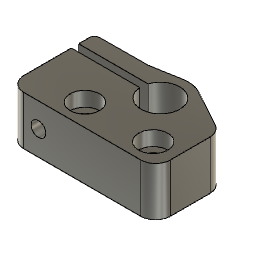
Y Axis Guide Rail Clamps (Autodesk Fusion 360 design; units mm, degrees)
Autodesk Fusion 360 part; units mm, degrees
sketch "Sketch4" plane through (0, 0, 0) normal (0, 0, 1) x (1, 0, 0)
  line L0 (-17.0224, 4.5069) -> (-7.2135, 4.5755)
  line L1 (-6.882, 4.6055) -> (-0.9889, 5.6389)
  line L2 (-18, 0) -> (-17.9997, 1.25) construction
  line L3 (-17.9997, 1.25) -> (-18.0154, 3.5)
  line L4 (-18, 0) -> (-18, -0.25) construction
  line L5 (-18, -0.25) -> (-3.9671, -0.25)
  line L6 (-17.9997, 1.25) -> (-3.7746, 1.2463)
  arc A0 (2.7555, 5.0182) -> (-0.9889, 5.6389) centre (0, 0) ccw
  arc A1 (-3.9671, -0.25) -> (-3.7746, 1.2463) centre (0, 0) ccw
  line L7 (-18, -0.25) -> (-18, -10)
  line L8 (-15, -13) -> (9, -13)
  line L9 (12, -10) -> (12, -1.8332)
  line L10 (10.444, 0.7965) -> (2.7555, 5.0182)
  arc A2 (-7.2135, 4.5755) -> (-6.882, 4.6055) centre (-7.2274, 6.5754) ccw
  arc A3 (-7.2135, 4.5755) -> (-6.882, 4.6055) centre (-7.2274, 6.5754) ccw
  arc A4 (12, -1.8332) -> (10.444, 0.7965) centre (9, -1.8332) ccw
  arc A5 (9, -13) -> (12, -10) centre (9, -10) ccw
  arc A6 (-18, -10) -> (-15, -13) centre (-15, -10) ccw
  arc A7 (-17.0224, 4.5069) -> (-18.0154, 3.5) centre (-17.0154, 3.507) ccw
  point P0 (-18.0224, 4.4999)
  dimension "d18" = 7.95
  dimension "d22" = 18
  dimension "d24" = 4.5
  dimension "d26" = 1.25
  dimension "d27" = 0.25
  dimension "d28" = 2
  dimension "d29" = 3
  dimension "d30" = 3
  dimension "d31" = 1
  dimension "d56" = 1.75
  constraint coincident A0.centre A1.centre
  constraint tangent L1 A0
  constraint perpendicular L0 L3
  constraint vertical L4
  constraint perpendicular L4 L5
  constraint perpendicular L2 L6
  constraint concentric A0 A1
  constraint tangent A0 L10
  constraint tangent L0 A2
  constraint tangent L1 A2
  constraint coincident L0 A2.start
  constraint coincident L1 A2.end
  constraint tangent L0 A3
  constraint tangent L1 A3
  constraint equal A2 A3
  constraint tangent L10 A4
  constraint tangent L9 A4
  constraint tangent L9 A5
  constraint tangent L8 A5
  constraint tangent L7 A6
  constraint tangent L8 A6
  constraint equal A5 A6
  constraint coincident P0 L3
  constraint coincident P0 L0
  constraint tangent L3 A7
  constraint tangent L0 A7
  measures "d18" diameter of A1
  measures "d22" distance of A0.centre L2.start
  measures "d24" distance of L2.start P0
  measures "d26" distance of L2.start L2.end
  measures "d27" distance of L2.start L4.end
  measures "d28" radius of A2
  measures "d29" radius of A4
  measures "d30" radius of A5
  measures "d31" radius of A7
  measures "d56" distance of A0 A1
extrude "Extrude2" add sketch "Sketch4" along normal blind 10 makes body 1
sketch "Sketch5" plane through (-0.0323, 4.6256, 0) normal (-0.006986, 0.999976, 0) x (-0.999976, -0.006986, 0)
  line L0 (7.1813, 0) -> (16.9905, 0)
  line L1 (16.9905, 0) -> (16.9905, 10)
  line L2 (16.9905, 10) -> (7.1813, 10)
  line L3 (7.1813, 10) -> (7.1813, 0)
  line L4 (12.0859, 10) -> (12.0859, 0) construction
  line L5 (16.9905, 5) -> (7.1813, 5) construction
  constraint midpoint L2 L4.start
  constraint midpoint L0 L4.end
  constraint midpoint L1 L5.start
  constraint midpoint L3 L5.end
hole "Hole2" at (-12.1179, 4.5412, 5) direction (0.006986, -0.999976, 0) diameter 3 end through all counterbore diameter 6 counterbore depth 2 bodies 1
sketch "Sketch6" plane through (0, 0, 10) normal (0, 0, 1) x (-1, 0, 0)
  line L0 (7.2135, -4.5755) -> (17.0224, -4.5069)
  arc A0 (17.0224, -4.5069) -> (18.0154, -3.5) centre (17.0154, -3.507) ccw
  line L1 (18.0154, -3.5) -> (17.9997, -1.25)
  line L2 (17.9997, -1.25) -> (3.7746, -1.2463)
  arc A1 (3.9671, 0.25) -> (3.7746, -1.2463) centre (0, 0) ccw
  line L3 (3.9671, 0.25) -> (18, 0.25)
  line L4 (18, 0.25) -> (18, 10)
  arc A2 (18, 10) -> (15, 13) centre (15, 10) ccw
  line L5 (15, 13) -> (-9, 13)
  arc A3 (-9, 13) -> (-12, 10) centre (-9, 10) ccw
  line L6 (-12, 10) -> (-12, 1.8332)
  arc A4 (-12, 1.8332) -> (-10.444, -0.7965) centre (-9, 1.8332) ccw
  line L7 (-10.444, -0.7965) -> (-2.7555, -5.0182)
  arc A5 (-2.7555, -5.0182) -> (0.9889, -5.6389) centre (0, 0) ccw
  line L8 (0.9889, -5.6389) -> (6.882, -4.6055)
  arc A6 (7.2135, -4.5755) -> (6.882, -4.6055) centre (7.2274, -6.5754) ccw
  line L9 (0, 0) -> (0, 3.975) construction
  line L10 (0, 3.975) -> (-12, 3.975) construction
  line L11 (-12, 3.975) -> (-12, 12.975) construction
  line L12 (-12, 8.475) -> (18, 8.475) construction
  line L13 (0, 3.975) -> (0, 13) construction
  line L14 (7, 8.475) -> (7, 6.4233) construction
  point P0 (-7, 8.475)
  point P1 (7, 8.475)
  dimension "d39" = 9
  dimension "d54" = 14
  dimension "d55" = 7
  constraint vertical L9
  constraint coincident A1.centre A5.centre
  constraint coincident L6 L10.end
  constraint tangent A1 L10
  constraint perpendicular L6 L10
  constraint perpendicular L10 L11
  constraint midpoint L11 L12.start
  constraint coincident L4 L12.end
  constraint perpendicular L4 L12
  constraint coincident L12 P0
  constraint coincident L12 P1
  constraint coincident L5 L13.end
  constraint perpendicular L5 L13
  constraint coincident P1 L14.start
  constraint perpendicular L12 L14
  measures "d39" distance of L10.end L11.end
  measures "d54" distance of P0 P1
  measures "d55" distance of L13 L14
hole "Hole3" at (7, -8.475, 10) direction (0, 0, -1) diameter 3 end through all counterbore diameter 6 counterbore depth 3 bodies 1
hole "Hole4" at (-7, -8.475, 10) direction (0, 0, -1) diameter 3 end through all counterbore diameter 6 counterbore depth 3 bodies 1
sketch "Sketch7" plane through (-18, 0, 0) normal (-1, 0, 0) x (0, -1, 0)
  line L0 (0.25, 0) -> (10, 0)
  line L1 (10, 0) -> (10, 10)
  line L2 (10, 10) -> (0.25, 10)
  line L3 (0.25, 10) -> (0.25, 0)
  line L4 (5.125, 10) -> (5.125, 0) construction
  line L5 (10, 5) -> (0.25, 5) construction
  line L6 (6, 7.875) -> (4.25, 7.875)
  line L7 (4.25, 7.875) -> (4.25, 2.125)
  line L8 (4.25, 2.125) -> (6, 2.125)
  line L9 (6, 2.125) -> (6, 7.875)
  line L10 (6, 7.875) -> (4.25, 2.125) construction
  line L11 (4.25, 7.875) -> (6, 2.125) construction
  point P0 (5.125, 5)
  dimension "d50" = 1.75
  dimension "d51" = 5.75
  constraint midpoint L2 L4.start
  constraint midpoint L0 L4.end
  constraint midpoint L1 L5.start
  constraint midpoint L3 L5.end
  constraint horizontal L6
  constraint perpendicular L6 L7
  constraint parallel L6 L8
  constraint parallel L7 L9
  constraint coincident L10 P0
  constraint coincident L11 P0
  constraint midpoint L4 P0
  measures "d50" distance of L7.end L8.end
  measures "d51" distance of L6.end L7.end
extrude "Extrude3" cut sketch "Sketch7" against normal blind 8.81 contours L6 L7 L8 L9 bodies 1
copy_body "Body->Comp1" bodies 1 removing the originals makes body 2 in component "Guide Rail Clamp 1st Direction"
component "Guide Rail Clamp 1st Direction" placed x (1, 0, 0) y (0, 1, 0) z (0, 0, 1) at (0, 0, 0)
